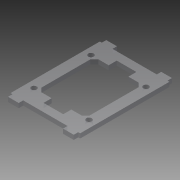
# Autodesk Inventor part: pcb_mount
Saved by Autodesk Inventor 2013 (Build 170138000, 138)
## iProperties
Created: 2014-05-23
Part Number: pcb_mount
Material: Polycarbonate, Clear
Document SubType Name: Modeling
Designer: balogh
Mass: 3.55442 g
Surface Area: 39.7277 cm^2
Volume: 3.97587 cm^3
Density: 0.894 g/cm^3
Author: balogh
Autodesk Inventor part; units mm, degrees
ref_plane "YZ Plane" through (0, 0, 0) normal (1, 0, 0) x (0, 1, 0)
ref_plane "XZ Plane" through (0, 0, 0) normal (0, 1, 0) x (-1, 0, 0)
ref_plane "XY Plane" through (0, 0, 0) normal (0, 0, 1) x (1, 0, 0)
sketch "Sketch1" plane through (0, 0, 0) normal (0, 0, 1) x (1, 0, 0)
  line L0 (-31.75, -21.2471) -> (-28.8544, -21.2471)
  line L1 (-28.8544, -21.2471) -> (-28.8544, -22.5171)
  line L2 (-28.8544, -22.5171) -> (28.8544, -22.5171)
  line L3 (28.8544, -22.5171) -> (28.8544, -21.2471)
  line L4 (28.8544, -21.2471) -> (31.75, -21.2471)
  line L5 (31.75, -21.2471) -> (31.75, -14.3129)
  line L6 (31.75, -14.3129) -> (28.8544, -14.3129)
  line L7 (28.8544, -14.3129) -> (28.8544, 14.3129)
  line L8 (28.8544, 14.3129) -> (31.75, 14.3129)
  line L9 (31.75, 14.3129) -> (31.75, 21.2471)
  line L10 (31.75, 21.2471) -> (28.8544, 21.2471)
  line L11 (28.8544, 21.2471) -> (28.8544, 22.5171)
  line L12 (28.8544, 22.5171) -> (-28.8544, 22.5171)
  line L13 (-28.8544, 22.5171) -> (-28.8544, 21.2471)
  line L14 (-28.8544, 21.2471) -> (-31.75, 21.2471)
  line L15 (-31.75, 21.2471) -> (-31.75, 14.3129)
  line L16 (-31.75, 14.3129) -> (-28.8544, 14.3129)
  line L17 (-28.8544, 14.3129) -> (-28.8544, -14.3129)
  line L18 (-28.8544, -14.3129) -> (-31.75, -14.3129)
  line L19 (-31.75, -14.3129) -> (-31.75, -21.2471)
  line L20 (18.415, -6.35) -> (23.6347, -6.35)
  line L21 (23.6347, -6.35) -> (23.6347, 6.35)
  line L22 (23.6347, 6.35) -> (18.415, 6.35)
  line L23 (18.415, 6.35) -> (18.415, 13.0429)
  line L24 (18.415, 13.0429) -> (15.875, 15.5829)
  line L25 (15.875, 15.5829) -> (-15.875, 15.5829)
  line L26 (-15.875, 15.5829) -> (-18.415, 13.0429)
  line L27 (-18.415, 13.0429) -> (-18.415, 6.35)
  line L28 (-18.415, 6.35) -> (-23.6347, 6.35)
  line L29 (-23.6347, 6.35) -> (-23.6347, -6.35)
  line L30 (-23.6347, -6.35) -> (-18.415, -6.35)
  line L31 (-18.415, -6.35) -> (-18.415, -13.0429)
  line L32 (-18.415, -13.0429) -> (-15.875, -15.5829)
  line L33 (-15.875, -15.5829) -> (15.875, -15.5829)
  line L34 (15.875, -15.5829) -> (18.415, -13.0429)
  line L35 (18.415, -13.0429) -> (18.415, -6.35)
  circle A0 centre (18.4151, -17.7801) radius 1.7526
  circle A1 centre (-18.415, 17.78) radius 1.7526
  circle A2 centre (-18.415, -17.78) radius 1.7526
  circle A3 centre (18.415, 17.78) radius 1.7526
  constraints: 72 end point, 21 parallel, 10 perpendicular, 4 centre point, 3 collinear, 3 equal radius
extrude "Extrusion1" add sketch "Sketch1" along normal blind 2.8956
body "Solid1"
